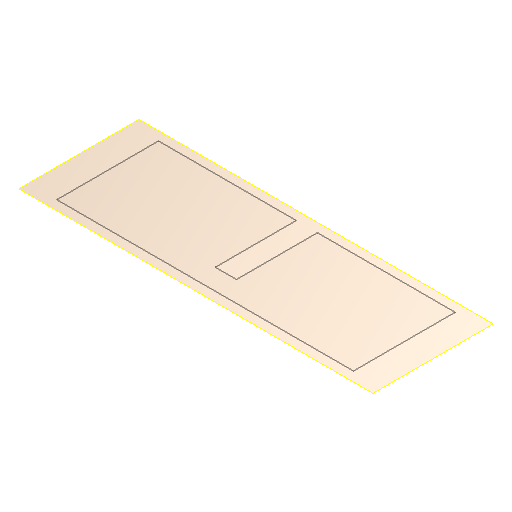
# Autodesk Inventor part: 00_coverglass_50x22
Saved by Autodesk Inventor 2024.1 (Build 281209000, 209)
## iProperties
Created: 2024-08-02
Part Number: 00_coverglass_50x22
Material: Generisch
Document SubType Name: Modeling
Designer: diederichbenedict
Density: 1 g/cm^3
Appearance: Polycarbonat - klar
Author: diederichbenedict
Autodesk Inventor part; units mm, degrees
ref_plane "YZ Plane" through (0, 0, 0) normal (1, 0, 0) x (0, 1, 0)
ref_plane "XZ Plane" through (0, 0, 0) normal (0, 1, 0) x (-1, 0, 0)
ref_plane "XY Plane" through (0, 0, 0) normal (0, 0, 1) x (1, 0, 0)
ref_plane "Arbeitsebene1" through (0, 0, 0.5) normal (0, 0, 1) x (1, 0, 0)
sketch "Skizze1" plane through (0, 0, 0.5) normal (0, 0, 1) x (1, 0, 0)
  circle A0 centre (12, 2.9) radius 1.5 projected
  circle A1 centre (-12, 2.9) radius 1.5 projected
  line L0 (2.5, 12.9) -> (2.5, -7.1) projected
  line L1 (2.5, -7.1) -> (2.25, -7.1) projected
  line L2 (2.25, -7.1) -> (2, -7.1) projected
  line L3 (2, -7.1) -> (1.75, -7.1) projected
  line L4 (1.75, -7.1) -> (1.5, -7.1) projected
  line L5 (1.5, -7.1) -> (1.25, -7.1) projected
  line L6 (1.25, -7.1) -> (1, -7.1) projected
  line L7 (1, -7.1) -> (0.75, -7.1) projected
  line L8 (0.75, -7.1) -> (0.5, -7.1) projected
  line L9 (0.5, -7.1) -> (0.25, -7.1) projected
  line L10 (0.25, -7.1) -> (0, -7.1) projected
  line L11 (0, -7.1) -> (-0.25, -7.1) projected
  line L12 (-0.25, -7.1) -> (-0.5, -7.1) projected
  line L13 (-0.5, -7.1) -> (-0.75, -7.1) projected
  line L14 (-0.75, -7.1) -> (-1, -7.1) projected
  line L15 (-1, -7.1) -> (-1.25, -7.1) projected
  line L16 (-1.25, -7.1) -> (-1.5, -7.1) projected
  line L17 (-1.5, -7.1) -> (-1.75, -7.1) projected
  line L18 (-1.75, -7.1) -> (-2, -7.1) projected
  line L19 (-2, -7.1) -> (-2.25, -7.1) projected
  line L20 (-2.25, -7.1) -> (-2.5, -7.1) projected
  line L21 (-2.5, -7.1) -> (-2.5, 12.9) projected
  line L22 (-2.5, 12.9) -> (-38, 12.9) projected
  line L23 (-38, 12.9) -> (-38, -12.9) projected
  line L24 (-38, -12.9) -> (38, -12.9) projected
  line L25 (38, -12.9) -> (38, 12.9) projected
  line L26 (38, 12.9) -> (2.5, 12.9) projected
  line L27 (35, -12) -> (-35, -12)
  line L28 (-35, -12) -> (-35, 12)
  line L29 (-35, 12) -> (35, 12)
  line L30 (35, 12) -> (35, -12)
  line L31 (35, -12) -> (-35, 12) construction
  line L32 (-35, -12) -> (35, 12) construction
  point P0 (0, 0)
  point P1 (-2.5, 12)
  point P2 (2.5, 12)
  dimension "d0" = 70
  dimension "d1" = 24
  constraints: 12 end point, 2 midpoint, 2 parallel, 1 horizontal, 1 perpendicular
  measures "d0" distance of L28.end L29.end
  measures "d1" distance of L27.end L28.end
extrude "Extrusion1" add sketch "Skizze1" along normal blind 0.15 contours A0 | A1 | L29 L30 L27 L28 L21 L20 L19 L18 L17 L16 L15 L14 L13 L12 L11 L10 L9 L8 L7 L6 L5 L4 L3 L2 L1 L0
